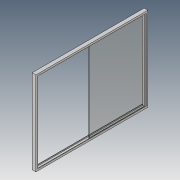
# Autodesk Inventor part: AVADemo_SlidingDoorFrame
Saved by Autodesk Inventor 2018.3 (Build 223284000, 284)
## iProperties
Created: 2019-11-06
Part Number: AVADemo_SlidingDoorFrame
Material: Generic
Document SubType Name: Modeling
Designer: MattBussey
Density: 1 g/cm^3
Appearance: Default
RuleStatus: InUse
Author: MattBussey
Autodesk Inventor part; units mm, degrees
ref_plane "YZ Plane" through (0, 0, 0) normal (1, 0, 0) x (0, 1, 0)
ref_plane "XZ Plane" through (0, 0, 0) normal (0, 1, 0) x (-1, 0, 0)
ref_plane "XY Plane" through (0, 0, 0) normal (0, 0, 1) x (1, 0, 0)
sketch "Sketch1" plane through (0, 0, 0) normal (1, 0, 0) x (0, 1, 0)
  line L0 (0, 0) -> (2286, 0)
  line L1 (2286, 0) -> (2286, -3048)
  line L2 (2286, -3048) -> (0, -3048)
  line L3 (0, -3048) -> (0, 0)
  line L4 (50.8, -50.8) -> (2235.2, -50.8)
  line L5 (2235.2, -50.8) -> (2235.2, -2997.2)
  line L6 (2235.2, -2997.2) -> (50.8, -2997.2)
  line L7 (50.8, -2997.2) -> (50.8, -50.8)
  point P0 (2235.2, -1524)
  point P1 (2286, -1524)
  point P2 (1143, -2997.2)
  point P3 (1143, -3048)
  dimension "d0" = 50.8
  dimension "d1" = 50.8
  dimension "d2" = 3048
  dimension "d3" = 2286
  constraints: 16 end point, 4 midpoint, 4 parallel, 2 horizontal, 2 perpendicular, 1 horizontal alignment, 1 vertical alignment
  measures "d0" distance between parallel lines of L2 L6
  measures "d1" distance between parallel lines of L1 L5
  measures "d2" distance of L0.end L1.end
  measures "d3" distance of L0.start L0.end
extrude "BaseFrame" add sketch "Sketch1" along normal blind 101.6
ref_plane "Work Plane1" through (50.8, 0, 0) normal (1, 0, 0) x (0, 0, -1)
sketch "Sketch2" plane through (50.8, 0, 0) normal (1, 0, 0) x (0, 0, -1)
  line L0 (0, 0) -> (0, 2286) construction
  line L1 (0, 2286) -> (3048, 2286) construction
  line L2 (3048, 2286) -> (3048, 0) construction
  line L3 (3048, 0) -> (0, 0) construction
  line L4 (3022.6, 2260.6) -> (25.4, 2260.6)
  line L5 (25.4, 2260.6) -> (25.4, 25.4) construction
  line L6 (25.4, 25.4) -> (3022.6, 25.4)
  line L7 (3022.6, 25.4) -> (3022.6, 2260.6) construction
  line L8 (2997.2, 50.8) -> (2997.2, 2235.2) projected
  line L9 (50.8, 2235.2) -> (50.8, 50.8) projected
  line L10 (50.8, 2235.2) -> (50.8, 2260.6)
  line L11 (2997.2, 2235.2) -> (2997.2, 2260.6)
  line L12 (2997.2, 50.8) -> (2997.2, 25.4)
  line L13 (50.8, 50.8) -> (50.8, 25.4)
  dimension "d6" = 25.4
  constraints: 16 end point, 6 point on line, 2 perpendicular, 3 other
  measures "d6" distance between parallel lines of L1 L4
extrude "DoorSlot" cut sketch "Sketch2" along normal mid plane 76.2
sketch "Sketch3" plane through (88.9, 0, 0) normal (-1, 0, 0) x (0, 0, 1)
  line L0 (-50.8, 25.4) -> (-2997.2, 25.4) projected
  line L1 (-2997.2, 2260.6) -> (-50.8, 2260.6) projected
  line L2 (-2997.2, 2260.6) -> (-1485.9, 2260.6)
  line L3 (-1485.9, 2260.6) -> (-1485.9, 25.4)
  line L4 (-1485.9, 25.4) -> (-2997.2, 25.4)
  line L5 (-2997.2, 25.4) -> (-2997.2, 2260.6)
  dimension "d9" = 1511.3
  constraints: 8 end point, 2 parallel, 1 horizontal, 1 perpendicular, 1 point on line
  measures "d9" distance between parallel lines of L5 L3
extrude "StationaryPanel" add sketch "Sketch3" along normal blind 38.1 separate body
ref_plane "Work Plane2" through (0, 0, -1524) normal (0, 0, 1) x (1, 0, 0)
mirror "MirrorRight" [suppressed]
mirror "MirrorRightExterior" [suppressed]
mirror "MirrorLeftExterior" [suppressed]
equation "\"d0\" = FrameWidth"
equation "\"d1\" = d0"
equation "\"d2\" = Width"
equation "\"d3\" = Height"
equation "\"d4\" = Depth"
equation "\"d6\" = 0.5 * FrameWidth"
equation "\"d7\" = 0.75 * Depth"
equation "\"d10\" = 0.375 * Depth"
equation "\"Width\" = 3048"
equation "\"Depth\" = 101.6"
equation "\"Height\" = 2286"
equation "\"FrameWidth\" = 50.8"
